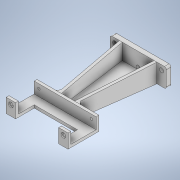
# Autodesk Inventor part: RL_spider_camera_mount
Saved by Autodesk Inventor 2022 (Build 260153000, 153)
## iProperties
Created: 2021-08-13
Part Number: RL_spider_camera_mount
Material: Generic
Document SubType Name: Modeling
Designer: Mock
Density: 1 g/cm^3
Appearance: Default
Author: Mock
Autodesk Inventor part; units mm, degrees
ref_plane "YZ Plane" through (0, 0, 0) normal (1, 0, 0) x (0, 1, 0)
ref_plane "XZ Plane" through (0, 0, 0) normal (0, 1, 0) x (-1, 0, 0)
sketch "Sketch1" plane through (0, 0, 0) normal (0, 0, 1) x (1, 0, 0)
  line L0 (0, 0) -> (40, 0)
  line L1 (40, 0) -> (40, 20)
  line L2 (40, 20) -> (0, 20)
  line L3 (0, 20) -> (0, 0)
  dimension "d69" = 20
  dimension "d70" = 40
  constraints: 8 end point, 2 parallel, 1 horizontal, 1 perpendicular, 1 other
  measures "d69" distance of L2.end L0.start
  measures "d70" distance of L0.start L0.end
extrude "Extrusion1" add sketch "Sketch1" along normal blind 5
sketch "Sketch2" plane through (0, 0, 5) normal (0, 0, 1) x (1, 0, 0)
  line L0 (40, 20) -> (0, 20) projected
  line L1 (0, 0) -> (40, 0) projected
  line L2 (0, 20) -> (40, 20)
  line L3 (40, 20) -> (40, 0)
  line L4 (40, 0) -> (0, 0)
  line L5 (0, 0) -> (0, 20)
  constraints: 8 end point, 2 parallel, 1 horizontal, 1 perpendicular
ref_plane "Work Plane1" through (0, 0, 80) normal (0, 0, 1) x (1, 0, 0)
sketch "Sketch3" plane through (0, 0, 80) normal (0, 0, 1) x (1, 0, 0)
  line L0 (10, 15) -> (30, 15)
  line L1 (30, 15) -> (30, 0)
  line L2 (30, 0) -> (10, 0)
  line L3 (10, 0) -> (10, 15)
  line L4 (0, 20) -> (0, 0) projected
  dimension "d71" = 20
  dimension "d72" = 15
  dimension "d73" = 10
  constraints: 8 end point, 2 parallel, 1 horizontal, 1 perpendicular
  measures "d71" distance of L0.start L0.end
  measures "d72" distance of L2.end L0.start
  measures "d73" distance between parallel lines of L3 L4
loft "Loft1" add profiles "Sketch3" section 2 edges at (40, 10, 5) (20, 20, 5) (0, 10, 5) (20, 0, 5)
sketch "Sketch4" plane through (0, 0, 80) normal (0, 0, 1) x (1, 0, 0)
  line L0 (53.025, 0) -> (-13.025, 0)
  line L1 (-13.025, 0) -> (-13.025, 15)
  line L2 (-13.025, 15) -> (53.025, 15)
  line L3 (53.025, 15) -> (53.025, 0)
  line L4 (30, 0) -> (10, 0) projected
  point P0 (0, 0)
  dimension "d16" = 66.05
  dimension "d18" = 15
  dimension "d76" = 0
  dimension "d78" = 13.025
  constraints: 8 end point, 2 parallel, 1 horizontal, 1 perpendicular
  measures "d16" distance of L0.start L0.end
  measures "d18" distance of L2.end L0.start
  measures "d76" distance between parallel lines of L0 L4
  measures "d78" distance from line of point (0, 0) L1
extrude "Extrusion2" add sketch "Sketch4" along normal blind 3
sketch "Sketch5" plane through (0, 0, 83) normal (0, 0, 1) x (1, 0, 0)
  line L0 (-13.025, 0) -> (53.025, 0) projected
  line L1 (-13.025, 15) -> (-13.025, 0) projected
  line L2 (53.025, 0) -> (-13.025, 0)
  line L3 (-13.025, 0) -> (-13.025, 3)
  line L4 (-13.025, 3) -> (53.025, 3)
  line L5 (53.025, 3) -> (53.025, 0)
  point P0 (0, 0)
  dimension "d22" = 3
  constraints: 8 end point, 2 parallel, 1 horizontal, 1 perpendicular, 1 point on line
  measures "d22" distance between parallel lines of L2 L4
extrude "Extrusion3" add sketch "Sketch5" along normal blind 27
sketch "Sketch6" plane through (0, 0, 110) normal (0, 0, 1) x (1, 0, 0)
  line L0 (53.025, 0) -> (53.025, 15) projected
  line L1 (-13.025, 15) -> (-13.025, 0) projected
  line L2 (53.025, 0) -> (-13.025, 0)
  line L3 (-13.025, 0) -> (-13.025, 15)
  line L4 (-13.025, 15) -> (53.025, 15)
  line L5 (53.025, 15) -> (53.025, 0)
  point P0 (0, 0)
  constraints: 8 end point, 2 parallel, 1 horizontal, 1 perpendicular
extrude "Extrusion4" add sketch "Sketch6" along normal blind 3
sketch "Sketch7" plane through (0, 0, 113) normal (0, 0, 1) x (1, 0, 0)
  circle A0 centre (-8.025, 10.5) radius 1.25
  circle A1 centre (48.025, 10.5) radius 1.25
  line L0 (53.025, 3) -> (-13.025, 3) projected
  line L1 (-13.025, 3) -> (53.025, 3) projected
  point P0 (0, 0)
  point P1 (20, 3)
  dimension "d27" = 7.5
  dimension "d28" = 7.5
  dimension "d29" = 56.05
  dimension "d30" = 28.025
  dimension "d31" = 2.5
  dimension "d32" = 2.5
  constraints: 2 centre point, 1 midpoint
  measures "d27" distance from line of A0.centre L0
  measures "d28" distance from line of A1.centre L0
  measures "d29" distance of A1.centre A0.centre
  measures "d30" horizontal distance of A0.centre point (20, 3)
  measures "d31" diameter of A0
  measures "d32" diameter of A1
extrude "Extrusion5" cut sketch "Sketch7" against normal blind 35
sketch "Sketch10" plane through (0, 0, 113) normal (0, 0, 1) x (1, 0, 0)
  circle A0 centre (48.025, 10.5) radius 1.25 projected
  circle A1 centre (48.025, 10.5) radius 2.5
  circle A2 centre (-8.025, 10.5) radius 1.25 projected
  circle A3 centre (-8.025, 10.5) radius 2.5
  point P0 (0, 0)
  dimension "d61" = 5
  dimension "d62" = 5
  constraints: 2 centre point, 2 coincident
  measures "d61" diameter of A1
  measures "d62" diameter of A3
extrude "Extrusion8" cut sketch "Sketch10" against normal blind 1
sketch "Sketch11" plane through (0, 0, 80) normal (0, 0, -1) x (-1, 0, 0)
  circle A0 centre (-48.025, 10.5) radius 1.25 projected
  circle A1 centre (-48.025, 10.5) radius 2.5
  circle A2 centre (8.025, 10.5) radius 1.25 projected
  circle A3 centre (8.025, 10.5) radius 2.5
  point P0 (0, 0)
  dimension "d65" = 5
  dimension "d66" = 5
  constraints: 2 centre point, 2 coincident
  measures "d65" diameter of A3
  measures "d66" diameter of A1
extrude "Extrusion9" cut sketch "Sketch11" against normal blind 1
sketch "Sketch12" plane through (-13.025, 15, 110) normal (0, 1, 0) x (1, 0, 0)
  line L0 (0, -3) -> (66.05, -3) projected
  line L1 (10, -3) -> (56.05, -3)
  line L2 (56.05, -3) -> (56.05, 17)
  line L3 (56.05, 17) -> (10, 17)
  line L4 (10, 17) -> (10, -3)
  line L5 (0, 27) -> (0, 0) projected
  line L6 (66.05, 27) -> (66.05, 0) projected
  line L7 (66.05, 27) -> (0, 27) projected
  point P0 (13.025, 110)
  dimension "d79" = 10
  dimension "d80" = 10
  dimension "d81" = 10
  constraints: 8 end point, 2 parallel, 1 horizontal, 1 perpendicular, 1 point on line
  measures "d79" distance between parallel lines of L4 L5
  measures "d80" distance between parallel lines of L6 L2
  measures "d81" distance between parallel lines of L7 L3
extrude "Extrusion10" cut sketch "Sketch12" against normal blind 15
sketch "Sketch15" plane through (0, 0, 0) normal (0, 0, -1) x (-1, 0, 0)
  line L0 (-30, 0) -> (-53.025, 0) projected
  line L1 (10, 20) -> (-50, 20)
  line L2 (-50, 20) -> (-50, 0)
  line L3 (-50, 0) -> (10, 0)
  line L4 (10, 0) -> (10, 20)
  line L5 (0, 20) -> (0, 0) projected
  line L6 (-40, 0) -> (-40, 20) projected
  dimension "d119" = 10
  dimension "d120" = 10
  constraints: 8 end point, 2 parallel, 1 horizontal, 1 perpendicular, 1 point on line
  measures "d119" distance between parallel lines of L4 L5
  measures "d120" distance between parallel lines of L6 L2
extrude "Extrusion13" add sketch "Sketch15" against normal blind 5 contours L0 L2 L1 L6 | L5 L1 L4 L3
fillet "Fillet1" radius 2 4 edges at (50, 20, 2.5) (50, 0, 2.5) (-10, 20, 2.5) (-10, 0, 2.5)
chamfer "Chamfer1" distance 3 angle 45 2 edges at (10, 7.5, 80) (30, 7.5, 80)
sketch "Sketch17" plane through (0, 20, 5) normal (0, 1, 0) x (1, 0, 0)
  line L0 (40, 0) -> (0, 0) projected
  line L1 (3.0265, 0) -> (13.0265, -75)
  line L2 (33, -75) -> (7, -75) projected
  line L3 (36.9735, 0) -> (26.9735, -75)
  line L4 (9.6035, -72.0263) -> (0, 0) projected
  line L5 (30.3965, -72.0263) -> (40, 0) projected
  point P0 (0, 5)
  dimension "d138" = 3
  dimension "d139" = 3
  constraints: 4 end point, 4 point on line, 2 parallel
  measures "d138" distance between parallel lines of L1 L4
  measures "d139" distance between parallel lines of L5 L3
extrude "Extrusion15" cut sketch "Sketch17" against normal blind 17
sketch "Sketch16" plane through (0, 0, 0) normal (0, 0, -1) x (-1, 0, 0)
  circle A0 centre (-45, 15) radius 2.2
  circle A1 centre (5, 15) radius 2.2
  circle A2 centre (-20, 5) radius 2.2
  line L0 (-50, 20) -> (-50, 0) projected
  line L1 (10, 20) -> (-50, 20) projected
  line L2 (10, 0) -> (10, 20) projected
  line L3 (-50, 0) -> (10, 0) projected
  point P0 (0, 0)
  dimension "d123" = 5
  dimension "d124" = 5
  dimension "d125" = 4.4
  dimension "d126" = 4.4
  dimension "d127" = 5
  dimension "d128" = 5
  dimension "d129" = 5
  dimension "d130" = 4.4
  dimension "d134" = 30
  constraints: 3 centre point
  measures "d123" distance from line of A0.centre L0
  measures "d124" distance from line of A0.centre L1
  measures "d125" diameter of A0
  measures "d126" diameter of A1
  measures "d127" distance from line of A1.centre L1
  measures "d128" distance from line of L2 A1.centre
  measures "d129" distance from line of L3 A2.centre
  measures "d130" diameter of A2
  measures "d134" distance from line of A2.centre L0
extrude "Extrusion16" cut sketch "Sketch16" against normal blind 6 contours A0 | A1 | A2
equation "\"d30\" = 0.5 * d29"
body "Solid1"
